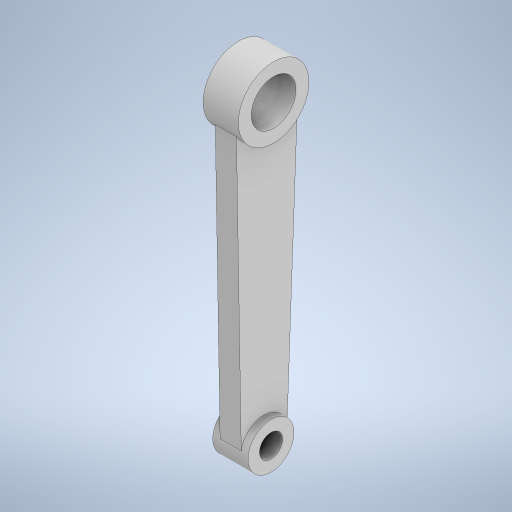
# Autodesk Inventor part: Handle
Saved by Autodesk Inventor 2023 (Build 270158000, 158)
## iProperties
Created: 2023-02-15
Part Number: Handle
Material: Generic
Document SubType Name: Modeling
Designer: deepa
Density: 1 g/cm^3
Appearance: Default
Author: deepa
Autodesk Inventor part; units mm, degrees
ref_plane "YZ Plane" through (0, 0, 0) normal (1, 0, 0) x (0, 1, 0)
ref_plane "XZ Plane" through (0, 0, 0) normal (0, 1, 0) x (-1, 0, 0)
ref_plane "XY Plane" through (0, 0, 0) normal (0, 0, 1) x (1, 0, 0)
sketch "Sketch1" plane through (0, 0, 0) normal (1, 0, 0) x (0, 1, 0)
  point P0 (0, 0)
sketch "Sketch2" plane through (0, 0, 0) normal (1, 0, 0) x (0, 1, 0)
  circle A0 centre (0, 0) radius 6.35
  circle A1 centre (0, 0) radius 10
  line L0 (-5.1891, 8.5483) -> (-85.1769, 7.1521)
  line L1 (-5.1891, 8.5483) -> (74.8109, 8.5483) construction
  circle A2 centre (-83.9993, 0.7508) radius 6.5088
  line L2 (-4.8085, -8.768) -> (-84.2461, -5.7533)
  circle A3 centre (-83.9993, 0.7508) radius 3.25
  point P0 (9.9976, 0.2197)
  point P1 (-4.8085, -8.768)
  point P2 (-5.1891, 8.5483)
  point P3 (-83.0459, 7.1893)
  dimension "d1" = 20
  dimension "d0" = 12.7
  dimension "d4" = 360
  dimension "d7" = 80
  dimension "d8" = 179
  dimension "d9" = 6.5
  constraints: 6 end point, 3 centre point, 3 coincident, 2 point on circle, 1 equal length, 1 horizontal, 1 tangent, 7 other
  measures "d0" diameter of A0
  measures "d7" distance of L0.start L0.end
  measures "d8" angle of L0 L1
  measures "d9" diameter of A3
extrude "Extrusion1" add sketch "Sketch2" along normal mid plane 10 contours A1 | A2 L0 | L0 A2
extrude "Extrusion2" add sketch "Sketch2" along normal mid plane 6 contours A1 L2 A2 L0 | A2 L0 picked at (-84.2044, 6.1062)
body "Solid1"
